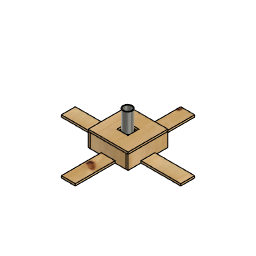
Test_Stand_v5 (Autodesk Fusion 360 design; units mm, degrees)
Autodesk Fusion 360 part; units mm, degrees
note: some values were not read from the file. Set by a fixed rule: which face or edge a step refers to.
sketch "Sketch1" plane through (0, 0, 0) normal (0, 0, 1) x (1, 0, 0) in component "Load Cell"
  line L0 (-37.5, 0) -> (37.5, 0)
  line L1 (37.5, 0) -> (37.5, -12.7)
  line L2 (37.5, -12.7) -> (-37.5, -12.7)
  line L3 (-37.5, -12.7) -> (-37.5, 0)
  line L4 (-37.5, -6.35) -> (37.5, -6.35) construction
  circle A0 centre (-22, -6.35) radius 2
  circle A1 centre (-32, -6.35) radius 2
  line L5 (0, 0) -> (0, -12.7) construction
  circle A2 centre (17.5, -6.35) radius 2
  circle A3 centre (32.5, -6.35) radius 2
  dimension "d1" = 75
  dimension "d2" = 12.7
  dimension "d3" = 4
  dimension "d4" = 4
  dimension "d5" = 22
  dimension "d6" = 10
  dimension "d7" = 4
  dimension "d8" = 4
  dimension "d10" = 15
  dimension "d54" = 5
  constraint horizontal L0
  constraint vertical L1
  constraint horizontal L2
  constraint vertical L3
  constraint midpoint L5.start L0
  constraint midpoint L3 L4.start
  constraint midpoint L1 L4.end
  constraint coincident L4 A0.centre
  constraint coincident L4 A1.centre
  constraint coincident L5.start origin
  constraint midpoint L2 L5.end
  constraint coincident L4 A2.centre
  constraint coincident L4 A3.centre
  measures "d1" distance of L0.start L0.end
  measures "d2" distance of L0.start L2.end
  measures "d3" diameter of A0
  measures "d4" diameter of A1
  measures "d5" distance of A0.centre L5
  measures "d6" distance of A0.centre A1.centre
  measures "d7" diameter of A2
  measures "d8" diameter of A3
  measures "d10" distance of A2.centre A3.centre
  measures "d54" distance of L1 A3.centre
extrude "Extrude1" add sketch "Sketch1" along normal blind 12.7 makes body 1 in component "Load Cell"
sketch "Sketch2" plane through (0, -12.7, 0) normal (0, -1, 0) x (1, 0, 0) in component "Load Cell"
  line L0 (-37.5, 0) -> (37.5, 0)
  line L1 (37.5, 0) -> (37.5, 12.7)
  line L2 (37.5, 12.7) -> (-37.5, 12.7)
  line L3 (-37.5, 12.7) -> (-37.5, 0)
  line L4 (-37.5, 6.35) -> (37.5, 6.35) construction
  circle A0 centre (-3, 6.35) radius 5.5
  circle A1 centre (3, 6.35) radius 5.5
  line L5 (0, 12.7) -> (0, 0) construction
  dimension "d13" = 11
  dimension "d14" = 11
  dimension "d15" = 3
  dimension "d16" = 3
  constraint midpoint L3 L4.start
  constraint midpoint L1 L4.end
  constraint coincident L4 A0.centre
  constraint coincident L4 A1.centre
  constraint midpoint L2 L5.start
  constraint coincident L5.end origin
  measures "d13" diameter of A1
  measures "d14" diameter of A0
  measures "d15" distance of A1.centre L5
  measures "d16" distance of A0.centre L5
extrude "Extrude2" cut sketch "Sketch2" against normal up to surface (12.7 mm away) contours A0 A1 | A0 A1 | A0 A1 bodies 1 in component "Load Cell"
sketch "Sketch1 (2)" plane through (0, 0, 12.7) normal (0, 0, 1) x (-1, 0, 0) in component "Stand"
  line L0 (-37.5, 12.7) -> (-37.5, 0)
  line L1 (-37.5, 0) -> (37.5, 0)
  line L2 (37.5, 0) -> (37.5, 12.7)
  line L3 (73, -93.65) -> (-127, -93.65)
  line L4 (-127, -93.65) -> (-127, 106.35)
  line L5 (-127, 106.35) -> (73, 106.35)
  line L6 (73, 106.35) -> (73, -93.65)
  line L7 (-27, -93.65) -> (-27, 106.35) construction
  line L8 (73, 6.35) -> (-127, 6.35) construction
  line L9 (-24, 6.35) -> (-30, 6.35) construction
  line L10 (0.5, -21.15) -> (-54.5, -21.15)
  line L11 (-54.5, -21.15) -> (-54.5, 33.85)
  line L12 (-54.5, 33.85) -> (0.5, 33.85)
  line L13 (0.5, 33.85) -> (0.5, -21.15)
  line L14 (0.5, 6.35) -> (-54.5, 6.35) construction
  line L15 (-27, -21.15) -> (-27, 33.85) construction
  dimension "d19" = 200
  dimension "d20" = 200
  dimension "d23" = 55
  dimension "d24" = 55
  constraint horizontal L3
  constraint vertical L4
  constraint horizontal L5
  constraint vertical L6
  constraint midpoint L3 L7.start
  constraint midpoint L5 L7.end
  constraint midpoint L6 L8.start
  constraint midpoint L4 L8.end
  constraint midpoint L8 L9
  constraint horizontal L10
  constraint vertical L11
  constraint horizontal L12
  constraint vertical L13
  constraint midpoint L13 L14.start
  constraint midpoint L11 L14.end
  constraint midpoint L10 L15.start
  constraint midpoint L12 L15.end
  constraint midpoint L9 L14
  measures "d19" distance of L3.start L5.end
  measures "d20" distance of L3.start L3.end
  measures "d23" distance of L10.end L11.end
  measures "d24" distance of L10.start L10.end
extrude "Extrude1'" add sketch "Sketch1 (2)" along normal blind 10 separate body makes body 2 in component "Stand"
sketch "Sketch2 (2)" plane through (0, 0, 12.7) normal (0, 0, -1) x (1, 0, 0) in component "Stand"
  line L0 (-0.5, 33.85) -> (54.5, 33.85)
  line L1 (54.5, 33.85) -> (54.5, -21.15)
  line L2 (54.5, -21.15) -> (-0.5, -21.15)
  line L3 (-0.5, -21.15) -> (-0.5, 33.85)
  line L4 (127, 106.35) -> (-73, 106.35)
  line L5 (-73, 106.35) -> (-73, -93.65)
  line L6 (-73, -93.65) -> (127, -93.65)
  line L7 (127, -93.65) -> (127, 106.35)
  line L8 (-73, 106.35) -> (-63, 106.35)
  line L9 (-63, 106.35) -> (-63, -93.65)
  line L10 (-63, -93.65) -> (-73, -93.65)
  line L11 (-73, -93.65) -> (-73, 106.35)
  dimension "d27" = 10
  constraint horizontal L8
  constraint vertical L9
  constraint horizontal L10
  constraint vertical L11
  constraint coincident L6 L9.end
  constraint coincident L4.end L5.start
  measures "d27" distance of L9.end L5.end
extrude "Extrude2'" add sketch "Sketch2 (2)" along normal blind 70 separate body contours L4 L5 L6 L8 L9 L10 L11 makes body 3 in component "Stand"
sketch "Sketch3" plane through (0, 0, 12.7) normal (0, 0, -1) x (1, 0, 0) in component "Stand"
  line L0 (-0.5, 33.85) -> (54.5, 33.85)
  line L1 (54.5, 33.85) -> (54.5, -21.15)
  line L2 (54.5, -21.15) -> (-0.5, -21.15)
  line L3 (-0.5, -21.15) -> (-0.5, 33.85)
  line L4 (127, 106.35) -> (-73, 106.35)
  line L5 (-73, 106.35) -> (-73, -93.65)
  line L6 (-73, -93.65) -> (127, -93.65)
  line L7 (127, -93.65) -> (127, 106.35)
  line L8 (117, 106.35) -> (117, -93.65)
  dimension "d30" = 10
  constraint coincident L4 L8.start
  constraint coincident L6 L8.end
  constraint perpendicular L6 L8
  measures "d30" distance of L7 L8
extrude "Extrude3" add sketch "Sketch3" along normal blind 70 separate body contours L4 L6 L7 L8 makes body 4 in component "Stand"
sketch "Sketch4" plane through (0, 0, 12.7) normal (0, 0, -1) x (1, 0, 0) in component "Stand"
  line L0 (-0.5, 33.85) -> (54.5, 33.85)
  line L1 (54.5, 33.85) -> (54.5, -21.15)
  line L2 (54.5, -21.15) -> (-0.5, -21.15)
  line L3 (-0.5, -21.15) -> (-0.5, 33.85)
  line L4 (127, 106.35) -> (-73, 106.35)
  line L5 (-73, 106.35) -> (-73, -93.65)
  line L6 (-73, -93.65) -> (127, -93.65)
  line L7 (127, -93.65) -> (127, 106.35)
  line L8 (-63, -93.65) -> (-63, 106.35)
  line L9 (117, 106.35) -> (117, -93.65)
  line L10 (-63, 96.35) -> (117, 96.35)
  dimension "d33" = 10
  constraint coincident L8 L10.start
  constraint coincident L9 L10.end
  constraint perpendicular L9 L10
  measures "d33" distance of L4 L10
extrude "Extrude4" add sketch "Sketch4" along normal blind 70 separate body contours L4 L8 L9 L10 makes body 5 in component "Stand"
sketch "Sketch5" plane through (0, 0, 12.7) normal (0, 0, -1) x (1, 0, 0) in component "Stand"
  line L0 (-0.5, 33.85) -> (54.5, 33.85)
  line L1 (54.5, 33.85) -> (54.5, -21.15)
  line L2 (54.5, -21.15) -> (-0.5, -21.15)
  line L3 (-0.5, -21.15) -> (-0.5, 33.85)
  line L4 (127, 106.35) -> (-73, 106.35)
  line L5 (-73, 106.35) -> (-73, -93.65)
  line L6 (-73, -93.65) -> (127, -93.65)
  line L7 (127, -93.65) -> (127, 106.35)
  line L8 (-63, -93.65) -> (-63, 106.35)
  line L9 (117, 106.35) -> (117, -93.65)
  line L10 (-63, -83.65) -> (117, -83.65)
  dimension "d36" = 10
  constraint coincident L8 L10.start
  constraint coincident L9 L10.end
  constraint perpendicular L9 L10
  measures "d36" distance of L6 L10
extrude "Extrude5" add sketch "Sketch5" along normal blind 70 separate body contours L6 L8 L9 L10 makes body 6 in component "Stand"
sketch "Sketch1 (3)" plane through (0, 0, 12.7) normal (0, 0, 1) x (-1, 0, 0) in component "Motor Holder"
  circle A0 centre (22, 6.35) radius 2
  circle A1 centre (-17.5, 6.35) radius 2
  circle A2 centre (32, 6.35) radius 2
  circle A3 centre (-32.5, 6.35) radius 2
  line L0 (37.5, 0) -> (37.5, 12.7)
  line L1 (-17.5, 6.35) -> (-32.5, 6.35) construction
  circle A4 centre (-25, 6.35) radius 23.5
  dimension "d40" = 47
  dimension "d55" = 7.5
  constraint coincident A1.centre L1.start
  constraint coincident A3.centre L1.end
  measures "d40" diameter of A4
  measures "d55" distance of A3.centre A4.centre
extrude "Extrude1''" add sketch "Sketch1 (3)" along normal blind 100 separate body contours A1 | A3 | A4 makes body 7 in component "Motor Holder"
shell "Shell1" thickness 4 removed faces 1 at (24.7209, -12.8194, 112.7) on bodies 7 in component "Motor Holder"
sketch "Sketch2 (3)" plane through (0, 0, 16.7) normal (0, 0, 1) x (-1, 0, 0) in component "Motor Holder"
  circle A0 centre (-25, 6.35) radius 19.5
  circle A1 centre (22, 6.35) radius 2
  circle A2 centre (-17.5, 6.35) radius 2
  circle A3 centre (32, 6.35) radius 2
  circle A4 centre (-32.5, 6.35) radius 2
  line L0 (37.5, 12.7) -> (-37.5, 12.7)
  line L1 (-37.5, 12.7) -> (-37.5, 0)
  line L2 (-37.5, 0) -> (37.5, 0)
  line L3 (37.5, 0) -> (37.5, 12.7)
extrude "Extrude2''" cut sketch "Sketch2 (3)" against normal up to surface (4 mm away) contours A2 | A4 bodies 7 in component "Motor Holder"
extrude "Extrude3'" add 1 faces at (24.5143, 1.1743, 16.7) along direction (0, 0, 1) blind 6 on bodies 7 bodies 7 in component "Motor Holder"
sketch "Sketch3 (2)" plane through (0, 0, 22.7) normal (0, 0, 1) x (-1, 0, 0) in component "Motor Holder"
  circle A0 centre (-17.5, 6.35) radius 2
  circle A1 centre (-32.5, 6.35) radius 2
  circle A2 centre (-25, 6.35) radius 19.5
  circle A3 centre (-32.5, 6.35) radius 4
  circle A4 centre (-17.5, 6.35) radius 4
  dimension "d48" = 8
  dimension "d49" = 8
  constraint concentric A1 A3
  constraint concentric A0 A4
  measures "d48" diameter of A3
  measures "d49" diameter of A4
fillet "Fillet1" radius 2 1 edges at (46.9097, 2.148, 12.7) on bodies 7 in component "Motor Holder"
sketch "Sketch6" plane through (0, -106.35, 0) normal (0, -1, 0) x (1, 0, 0) in component "Stand"
  line L0 (117, 12.7) -> (-63, 12.7)
  line L1 (-63, 12.7) -> (-63, -57.3)
  line L2 (-63, -57.3) -> (117, -57.3)
  line L3 (117, -57.3) -> (117, 12.7)
  line L4 (-8, -57.3) -> (-8, -47.3)
  line L5 (-8, -47.3) -> (62, -47.3)
  line L6 (62, -47.3) -> (62, -57.3)
  dimension "d56" = 70
  dimension "d57" = 10
  dimension "d58" = 55
  dimension "d59" = 55
  constraint coincident L2 L4.start
  constraint perpendicular L2 L4
  constraint perpendicular L4 L5
  constraint coincident L2 L6.end
  constraint perpendicular L2 L6
  measures "d56" distance of L4.end L5.end
  measures "d57" distance of L4.start L4.end
  measures "d58" distance of L1 L4
  measures "d59" distance of L3 L6
extrude "Extrude6" cut sketch "Sketch6" against normal up to surface (200 mm away) contours L2 L4 L5 L6 bodies 5 6 in component "Stand"
sketch "Sketch7" plane through (127, 0, 0) normal (1, 0, 0) x (0, 1, 0) in component "Stand"
  line L0 (93.65, 12.7) -> (-106.35, 12.7)
  line L1 (-106.35, 12.7) -> (-106.35, -57.3)
  line L2 (-106.35, -57.3) -> (93.65, -57.3)
  line L3 (93.65, -57.3) -> (93.65, 12.7)
  line L4 (-41.35, -57.3) -> (-41.35, -47.3)
  line L5 (-41.35, -47.3) -> (28.65, -47.3)
  line L6 (28.65, -47.3) -> (28.65, -57.3)
  dimension "d62" = 70
  dimension "d63" = 10
  dimension "d64" = 65
  dimension "d65" = 65
  constraint coincident L2 L4.start
  constraint perpendicular L2 L4
  constraint perpendicular L4 L5
  constraint coincident L2 L6.end
  constraint perpendicular L2 L6
  measures "d62" distance of L4.end L5.end
  measures "d63" distance of L4.start L4.end
  measures "d64" distance of L1 L4
  measures "d65" distance of L3 L6
extrude "Extrude7" cut sketch "Sketch7" against normal up to surface (200 mm away) contours L2 L4 L5 L6 bodies 3 4 in component "Stand"
sketch "Sketch1 (4)" plane through (0, 0, -47.3) normal (0, 0, -1) x (1, 0, 0) in component "Legs"
  line L0 (62, -83.65) -> (-8, -83.65)
  line L1 (-8, -83.65) -> (-8, -93.65)
  line L2 (-8, -93.65) -> (62, -93.65)
  line L3 (62, -93.65) -> (62, -83.65)
  line L4 (117, 41.35) -> (117, -28.65)
  line L5 (117, -28.65) -> (127, -28.65)
  line L6 (127, -28.65) -> (127, 41.35)
  line L7 (127, 41.35) -> (117, 41.35)
  line L8 (-8, 96.35) -> (62, 96.35)
  line L9 (62, 96.35) -> (62, 106.35)
  line L10 (62, 106.35) -> (-8, 106.35)
  line L11 (-8, 106.35) -> (-8, 96.35)
  line L12 (-63, -28.65) -> (-63, 41.35)
  line L13 (-63, 41.35) -> (-73, 41.35)
  line L14 (-73, 41.35) -> (-73, -28.65)
  line L15 (-73, -28.65) -> (-63, -28.65)
  line L16 (62, -28.65) -> (327, -28.65)
  line L17 (327, -28.65) -> (327, 41.35)
  line L18 (327, 41.35) -> (62, 41.35)
  line L19 (127, -93.65) -> (127, -28.65)
  line L20 (62, -28.65) -> (62, -293.65)
  line L21 (62, -293.65) -> (-8, -293.65)
  line L22 (-8, -293.65) -> (-8, -28.65)
  line L23 (-8, -28.65) -> (-273, -28.65)
  line L24 (-273, -28.65) -> (-273, 41.35)
  line L25 (-273, 41.35) -> (-8, 41.35)
  line L26 (62, 41.35) -> (62, 306.35)
  line L27 (62, 306.35) -> (-8, 306.35)
  line L28 (-8, 306.35) -> (-8, 41.35)
  dimension "d68" = 70
  dimension "d70" = 200
  dimension "d71" = 70
  dimension "d72" = 200
  dimension "d73" = 70
  dimension "d76" = 200
  dimension "d77" = 70
  dimension "d78" = 200
  constraint perpendicular L6 L16
  constraint perpendicular L16 L17
  constraint perpendicular L4 L18
  constraint perpendicular L16 L20
  constraint perpendicular L20 L21
  constraint perpendicular L21 L22
  constraint perpendicular L12 L23
  constraint perpendicular L23 L24
  constraint perpendicular L24 L25
  constraint coincident L12.start L23
  constraint coincident L22.end L23.start
  constraint coincident L2.end L20
  constraint perpendicular L10 L26
  constraint perpendicular L26 L27
  constraint perpendicular L8 L28
  constraint coincident L8.start L28
  constraint coincident L25.end L28.end
  constraint coincident L4.start L18
  constraint coincident L18.end L26.start
  measures "d68" distance of L16.end L17.end
  measures "d70" distance of L16.end L19
  measures "d71" distance of L20.end L21.end
  measures "d72" distance of L2.end L20.end
  measures "d73" distance of L23.end L24.end
  measures "d76" distance of L13.end L24.end
  measures "d77" distance of L26.end L27.end
  measures "d78" distance of L10.end L27.end
extrude "Extrude1'''" add sketch "Sketch1 (4)" along normal blind 10 separate body makes body 8 in component "Legs"
component "Load Cell" placed x (1, 0, 0) y (0, 1, 0) z (0, 0, 1) at (0, 0, 0)
component "Stand" placed x (1, 0, 0) y (0, 1, 0) z (0, 0, 1) at (0, 0, 0)
component "Motor Holder" placed x (1, 0, 0) y (0, 1, 0) z (0, 0, 1) at (0, 0, 0)
component "Legs" placed x (1, 0, 0) y (0, 1, 0) z (0, 0, 1) at (0, 0, 0)
